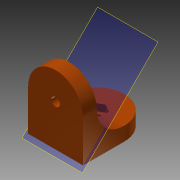
# Autodesk Inventor part: edge tab
Saved by Autodesk Inventor 2013 (Build 170138000, 138)
## iProperties
Created: 2013-07-28
Part Number: edge tab
Material: Generic
Document SubType Name: Modeling
Designer: employee
Density: 1 g/cm^3
Mass: 4.32348 g
Surface Area: 22.6905 cm^2
Volume: 4.32348 cm^3
Author: employee
Autodesk Inventor part; units mm, degrees
ref_plane "YZ Plane" through (0, 0, 0) normal (1, 0, 0) x (0, 1, 0)
ref_plane "XZ Plane" through (0, 0, 0) normal (0, 1, 0) x (-1, 0, 0)
ref_plane "XY Plane" through (0, 0, 0) normal (0, 0, 1) x (1, 0, 0)
sketch "Sketch1" plane through (0, 0, 0) normal (0, 0, 1) x (1, 0, 0)
  line L0 (0, 0) -> (20, 0)
  line L1 (20, 0) -> (20, 25)
  line L2 (20, 25) -> (0, 25)
  line L3 (0, 25) -> (0, 0)
  dimension "d0" = 20
  dimension "d2" = 25
  constraints: 8 end point, 2 parallel, 1 coincident, 1 horizontal, 1 perpendicular
  measures "d0" distance of L0.start L0.end
  measures "d2" distance of L2.end L0.start
extrude "Extrusion1" add sketch "Sketch1" along normal blind 5
sketch "Sketch2" plane through (0, 0, 5) normal (0, 0, 1) x (1, 0, 0)
  line L0 (0, 0) -> (20, 0) projected
  line L1 (20, 0) -> (20, 25) projected
  line L2 (0, 25) -> (0, 0) projected
  line L3 (0, 0) -> (20, 0)
  line L4 (20, 0) -> (20, 5)
  line L5 (20, 5) -> (0, 5)
  line L6 (0, 5) -> (0, 0)
  dimension "d5" = 5
  constraints: 8 end point, 3 point on line, 2 parallel, 1 horizontal, 1 perpendicular
  measures "d5" distance between parallel lines of L0 L5
extrude "Extrusion2" add sketch "Sketch2" along normal blind 20
sketch "Sketch3" plane through (0, 5, 5) normal (0, 1, 0) x (1, 0, 0)
  line L0 (20, -20) -> (0, -20) projected
  line L1 (20, 0) -> (20, -20) projected
  circle A0 centre (10, -10) radius 1.55
  point P0 (0, 5)
  point P1 (20, -10)
  point P2 (10, -20)
  dimension "d8" = 3.1
  constraints: 2 midpoint, 1 centre point, 1 horizontal alignment, 1 vertical alignment
  measures "d8" diameter of A0
extrude "Extrusion3" cut sketch "Sketch3" against normal through all
sketch "Sketch4" plane through (0, 5, 5) normal (0, 1, 0) x (1, 0, 0)
  circle A0 centre (10, -10) radius 1.55 projected
  line L0 (10, -13.2332) -> (7.2, -11.6166)
  line L1 (7.2, -11.6166) -> (7.2, -8.3834)
  line L2 (7.2, -8.3834) -> (10, -6.7668)
  line L3 (10, -6.7668) -> (12.8, -8.3834)
  line L4 (12.8, -8.3834) -> (12.8, -11.6166)
  line L5 (12.8, -11.6166) -> (10, -13.2332)
  point P0 (0, 5)
  dimension "d12" = 5.6
  constraints: 12 end point, 1 coincident, 1 vertical, 13 other
  measures "d12" distance between parallel lines of L4 L1
extrude "Extrusion4" cut sketch "Sketch4" against normal blind 2.5
ref_plane "Work Plane1" through (15, 5, 5) normal (0, 0.7071068, -0.7071068) x (1, 0, 0)
mirror "Mirror1" about plane through (15, 5, 5) normal (0, 0.7071068, -0.7071068) of "Extrusion4", "Extrusion3"
fillet "Fillet1" radius 10 4 edges at (0, 25, 2.5) (20, 25, 2.5) (20, 2.5, 25) (0, 2.5, 25)
fillet "Fillet2" radius 10 1 edges at (10, 5, 5)
body "Solid1"
